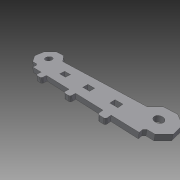
# Autodesk Inventor part: rope_mount_b
Saved by Autodesk Inventor 2014 (Build 180170000, 170)
## iProperties
Created: 2013-12-16
Part Number: rope_mount_b
Material: Generic
Document SubType Name: Modeling
Designer: buben
Density: 1 g/cm^3
Appearance: Default
Author: buben
Autodesk Inventor part; units mm, degrees
ref_plane "YZ Plane" through (0, 0, 0) normal (1, 0, 0) x (0, 1, 0)
ref_plane "XZ Plane" through (0, 0, 0) normal (0, 1, 0) x (-1, 0, 0)
ref_plane "XY Plane" through (0, 0, 0) normal (0, 0, 1) x (1, 0, 0)
sketch "Sketch1" plane through (0, 0, 0) normal (0, 0, 1) x (1, 0, 0)
  circle A0 centre (-2, 20.4853) radius 4.25
  circle A1 centre (124.1, 20.4853) radius 4.25
  line L0 (-17, 26.4853) -> (-17, 14.4853)
  line L1 (-17, 26.4853) -> (-8.5147, 34.9706)
  line L2 (-17, 14.4853) -> (-8.5147, 6)
  line L3 (-8.5147, 34.9706) -> (130.6147, 34.9706)
  line L4 (130.6147, 34.9706) -> (139.1, 26.4853)
  line L5 (139.1, 26.4853) -> (139.1, 14.4853)
  line L6 (139.1, 14.4853) -> (130.6147, 6)
  circle A2 centre (-2, 20.4853) radius 13 construction
  circle A3 centre (-2, 20.4853) radius 17 construction
  line L7 (-8.5147, 6) -> (0, 6)
  line L8 (0, 6) -> (0, 0)
  line L9 (130.6147, 6) -> (122.1, 6)
  line L10 (122.1, 6) -> (122.1, 0)
  line L11 (122.1, 0) -> (0, 0)
  point P0 (0, 0)
  point P1 (-17, 20.4853)
  dimension "d0" = 8.5
  dimension "d1" = 126.1
  dimension "d2" = 45
  dimension "d3" = 12
  dimension "d4" = 26
  dimension "d5" = 34
  dimension "d6" = 15
  dimension "d7" = 6
  dimension "d10" = 15
  dimension "d18" = 2
  constraints: 24 end point, 8 perpendicular, 4 centre point, 4 equal length, 4 horizontal alignment, 3 coincident, 2 parallel, 1 equal radius, 1 midpoint, 1 vertical
  measures "d0" diameter of A0
  measures "d1" distance of A1.centre A0.centre
  measures "d2" angle of L0 L1
  measures "d3" distance of L0.start L0.end
  measures "d4" diameter of A2
  measures "d5" diameter of A3
  measures "d6" distance from line of A0.centre L0
  measures "d7" distance of L7.end L8.end
  measures "d10" distance from line of L5 A1.centre
  measures "d18" distance from line of L10 A1.centre
extrude "Extrusion1" add sketch "Sketch1" along normal blind 6
sketch "Sketch2" plane through (0, 0, 6) normal (0, 0, 1) x (1, 0, 0)
  line L0 (130.6147, 34.9706) -> (-8.5147, 34.9706) projected
  line L1 (-8.5147, 34.9706) -> (-17, 26.4853) projected
  line L2 (3.4853, 34.9706) -> (11.9706, 26.4853)
  line L3 (11.9706, 26.4853) -> (110.1294, 26.4853)
  line L4 (110.1294, 26.4853) -> (118.6147, 34.9706)
  point P0 (-17, 14.4853)
  dimension "d13" = 12
  dimension "d14" = 12
  dimension "d15" = 12
  constraints: 6 end point, 2 perpendicular, 2 point on line, 1 horizontal alignment, 1 parallel
  measures "d13" distance of L1.end point (-17, 14.485)
  measures "d14" distance of L2.start L0.end
  measures "d15" distance of L0.start L4.end
extrude "Extrusion2" cut sketch "Sketch2" against normal blind 6
sketch "Sketch3" plane through (0, 0, 6) normal (0, 0, 1) x (1, 0, 0)
  line L0 (0, 0) -> (122.1, 0) projected
  line L1 (110.1294, 26.4853) -> (11.9706, 26.4853) projected
  line L2 (57.05, 16) -> (65.05, 16)
  line L3 (65.05, 16) -> (65.05, 10)
  line L4 (65.05, 10) -> (57.05, 10)
  line L5 (57.05, 10) -> (57.05, 16)
  line L6 (27.05, 16) -> (35.05, 16)
  line L7 (35.05, 16) -> (35.05, 10)
  line L8 (35.05, 10) -> (27.05, 10)
  line L9 (27.05, 10) -> (27.05, 16)
  line L10 (87.05, 16) -> (95.05, 16)
  line L11 (95.05, 16) -> (95.05, 10)
  line L12 (95.05, 10) -> (87.05, 10)
  line L13 (87.05, 10) -> (87.05, 16)
  point P0 (61.05, 16)
  point P1 (61.05, 26.4853)
  dimension "d20" = 8
  dimension "d21" = 6
  dimension "d22" = 8
  dimension "d23" = 8
  dimension "d24" = 10
  dimension "d25" = 22
  dimension "d26" = 22
  constraints: 24 end point, 6 parallel, 4 collinear, 3 horizontal, 3 perpendicular, 2 midpoint, 1 vertical alignment
  measures "d20" distance of L6.start L6.end
  measures "d21" distance of L8.end L6.start
  measures "d22" distance of L2.start L2.end
  measures "d23" distance of L10.start L10.end
  measures "d24" distance between parallel lines of L0 L8
  measures "d25" distance between parallel lines of L5 L7
  measures "d26" distance between parallel lines of L13 L3
extrude "Extrusion3" cut sketch "Sketch3" against normal through all
sketch "Sketch4" plane through (0, 0, 6) normal (0, 0, 1) x (1, 0, 0)
  line L0 (0, 0) -> (122.1, 0) projected
  line L1 (13.1, 0) -> (21.1, 0)
  line L2 (21.1, 0) -> (21.1, -4)
  line L3 (19.1, -6) -> (15.1, -6)
  line L4 (13.1, -4) -> (13.1, 0)
  line L5 (51.1, 0) -> (59.1, 0)
  line L6 (59.1, 0) -> (59.1, -4)
  line L7 (57.1, -6) -> (53.1, -6)
  line L8 (51.1, -4) -> (51.1, 0)
  line L9 (89.1, 0) -> (97.1, 0)
  line L10 (97.1, 0) -> (97.1, -4)
  line L11 (95.1, -6) -> (91.1, -6)
  line L12 (89.1, -4) -> (89.1, 0)
  arc A0 (13.1, -4) -> (15.1, -6) centre (15.1, -4) ccw
  arc A1 (19.1, -6) -> (21.1, -4) centre (19.1, -4) ccw
  arc A2 (51.1, -4) -> (53.1, -6) centre (53.1, -4) ccw
  arc A3 (57.1, -6) -> (59.1, -4) centre (57.1, -4) ccw
  arc A4 (89.1, -4) -> (91.1, -6) centre (91.1, -4) ccw
  arc A5 (95.1, -6) -> (97.1, -4) centre (95.1, -4) ccw
  dimension "d29" = 2
  dimension "d30" = 8
  dimension "d31" = 8
  dimension "d32" = 8
  dimension "d33" = 6
  dimension "d34" = 6
  dimension "d35" = 6
  dimension "d36" = 25
  dimension "d37" = 30
  dimension "d38" = 30
  constraints: 24 end point, 12 point on circle, 12 tangent, 6 centre point, 6 parallel, 5 equal radius, 3 horizontal, 3 perpendicular, 3 point on line
  measures "d29" radius of A0
  measures "d30" distance between parallel lines of L2 L4
  measures "d31" distance between parallel lines of L6 L8
  measures "d32" distance between parallel lines of L10 L12
  measures "d33" distance between parallel lines of L3 L1
  measures "d34" distance between parallel lines of L7 L5
  measures "d35" distance between parallel lines of L11 L9
  measures "d36" distance from line of L0.end L10
  measures "d37" distance between parallel lines of L12 L6
  measures "d38" distance between parallel lines of L2 L8
extrude "Extrusion4" add sketch "Sketch4" against normal blind 6
chamfer "Chamfer1" distance 2 angle 45 2 edges at (0, 6, 3) (122.1, 6, 3)
equation "\"d14\" = d13"
equation "\"d15\" = d14"
equation "\"d26\" = d25"
body "Solid1"
